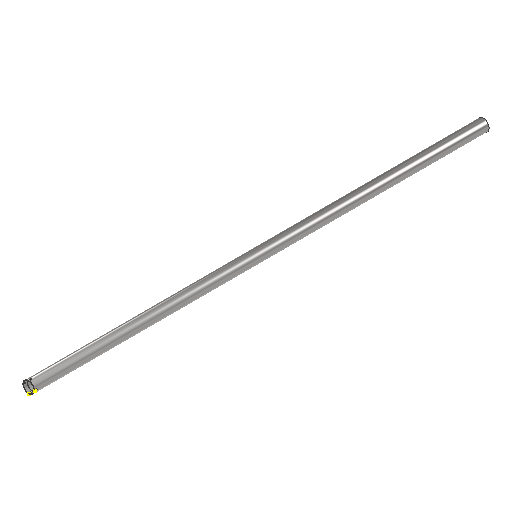
# Autodesk Inventor part: B_probe_pipe_5_for-non-rotating_1
Saved by Autodesk Inventor 2026.2 (Build 302298000, 298)
## iProperties
Created: 2026-01-05
Part Number: B_probe_pipe_5_for-non-rotating_1
Material: ステンレス鋼 440C
Document SubType Name: Sheet Metal
Designer: 水野 薫哉
Density: 7.75 g/cm^3
Sheet Metal Rule: Default
Appearance: 半つや出し
Author: 水野 薫哉
Autodesk Inventor part; units mm, degrees
ref_plane "XY Plane" through (0, 0, 0) normal (0, 0, 1) x (1, 0, 0)
sketch "スケッチ1" plane through (0, 0, 0) normal (0, 0, 1) x (1, 0, 0)
  circle A0 centre (0, 0) radius 17
  circle A1 centre (0, 0) radius 13.6
  dimension "d0" = 34
  dimension "d1" = 27.2
  constraints: 2 centre point, 2 coincident
  measures "d0" diameter of A0
  measures "d1" diameter of A1
extrude "押し出し1" add sketch "スケッチ1" against normal blind 1300
sketch "スケッチ3" plane through (0, 0, 0) normal (0, 0, 1) x (1, 0, 0)
  circle A0 centre (0, 0) radius 15
  dimension "d8" = 30
  constraints: 1 centre point, 1 coincident
  measures "d8" diameter of A0
extrude "押し出し3" cut sketch "スケッチ3" against normal blind 10
ref_plane "作業平面6" through (17, 0, 0) normal (1, 0, 0) x (0, 1, 0)
ref_plane "作業平面7" through (-17, 0, 0) normal (1, 0, 0) x (0, 1, 0)
sketch "スケッチ14" plane through (17, 0, 0) normal (1, 0, 0) x (0, 1, 0)
  point P0 (0, 0)
sketch "スケッチ15" plane through (17, 0, 0) normal (1, 0, 0) x (0, 1, 0)
  circle A0 centre (0, -5) radius 1.15
  point P0 (0, 0)
  dimension "d54" = 2.3
  dimension "d55" = 5
  constraints: 1 centre point
  measures "d54" diameter of A0
  measures "d55" distance of point (0, 0) A0.centre
ref_plane "作業平面8" through (0, 17, 0) normal (0, 1, 0) x (-1, 0, 0)
ref_plane "作業平面9" through (0, -17, 0) normal (0, 1, 0) x (-1, 0, 0)
sketch "スケッチ16" plane through (0, 17, 0) normal (0, 1, 0) x (-1, 0, 0)
  circle A0 centre (0, -5) radius 1.15
  point P0 (0, 0)
  dimension "d58" = 2.3
  dimension "d59" = 5
  constraints: 1 centre point
  measures "d58" diameter of A0
  measures "d59" distance of point (0, 0) A0.centre
extrude "押し出し13" cut sketch "スケッチ15" against normal through all
extrude "押し出し14" cut sketch "スケッチ16" against normal through all
sketch "スケッチ19" plane through (17, 0, 0) normal (1, 0, 0) x (0, 1, 0)
  circle A0 centre (0, -5) radius 2.1
  line L0 (17, 0) -> (-17, 0) projected
  point P0 (0, 0)
  dimension "d64" = 4.2
  dimension "d65" = 5
  constraints: 1 centre point
  measures "d64" diameter of A0
  measures "d65" distance from line of L0 A0.centre
extrude "押し出し15" cut sketch "スケッチ19" against normal blind 1
sketch "スケッチ20" plane through (0, 17, 0) normal (0, 1, 0) x (-1, 0, 0)
  circle A0 centre (0, -5) radius 2.1
  line L0 (17, 0) -> (-17, 0) projected
  point P0 (0, 0)
  dimension "d68" = 4.2
  dimension "d69" = 5
  constraints: 1 centre point
  measures "d68" diameter of A0
  measures "d69" distance from line of L0 A0.centre
extrude "押し出し16" cut sketch "スケッチ20" against normal blind 1
sketch "スケッチ21" plane through (-17, 0, 0) normal (1, 0, 0) x (0, 1, 0)
  circle A0 centre (0, -5) radius 2.1
  line L0 (17, 0) -> (-17, 0) projected
  point P0 (0, 0)
  dimension "d72" = 4.2
  dimension "d73" = 5
  constraints: 1 centre point
  measures "d72" diameter of A0
  measures "d73" distance from line of L0 A0.centre
extrude "押し出し17" cut sketch "スケッチ21" along normal blind 1
sketch "スケッチ22" plane through (0, -17, 0) normal (0, 1, 0) x (-1, 0, 0)
  point P0 (0, 0)
sketch "スケッチ23" plane through (0, -17, 0) normal (0, 1, 0) x (-1, 0, 0)
  circle A0 centre (0, -5) radius 2.1
  line L0 (17, 0) -> (-17, 0) projected
  point P0 (0, 0)
  dimension "d76" = 4.2
  dimension "d77" = 5
  constraints: 1 centre point
  measures "d76" diameter of A0
  measures "d77" distance from line of L0 A0.centre
extrude "押し出し18" cut sketch "スケッチ23" along normal blind 1
equation "\"BendRadius\" = Thickness"
equation "\"BendReliefWidth\" = Thickness"
equation "\"BendReliefDepth\" = 0.5 * Thickness"
equation "\"CornerReliefSize\" = 4 * Thickness"
equation "\"MinimumRemnant\" = 2 * Thickness"
equation "\"TransitionRadius\" = BendRadius"
equation "\"JacobiRadiusSize\" = BendRadius"
equation "\"GapSize\" = Thickness"
equation "\"Thickness\" = 3.048"
